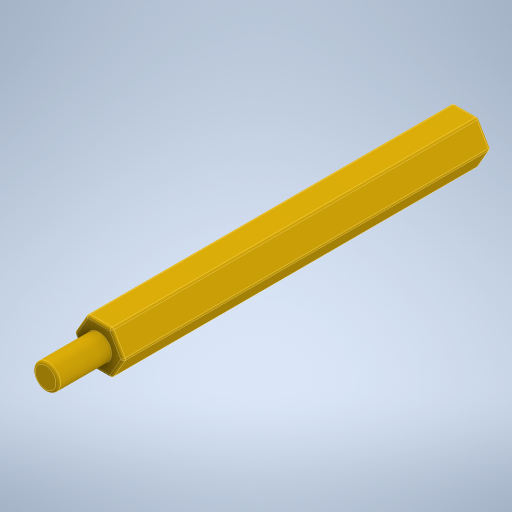
# Autodesk Inventor part: Espaciador_40mm
Saved by Autodesk Inventor 2023 (Build 270158030, 158C)
## iProperties
Created: 2022-07-21
Part Number: Espaciador_40mm
Material: Genérico
Document SubType Name: Modeling
Designer: luisn
Density: 1 g/cm^3
Appearance: Valor por defecto
Author: luisn
Autodesk Inventor part; units mm, degrees
ref_plane "YZ Plane" through (0, 0, 0) normal (1, 0, 0) x (0, 1, 0)
ref_plane "XZ Plane" through (0, 0, 0) normal (0, 1, 0) x (-1, 0, 0)
ref_plane "XY Plane" through (0, 0, 0) normal (0, 0, 1) x (1, 0, 0)
sketch "Boceto1" plane through (0, 0, 0) normal (0, 0, 1) x (1, 0, 0)
  line L0 (1.3423, 2.325) -> (2.6847, 0)
  line L1 (2.6847, 0) -> (1.3423, -2.325)
  line L2 (1.3423, -2.325) -> (-1.3423, -2.325)
  line L3 (-1.3423, -2.325) -> (-2.6847, 0)
  line L4 (-2.6847, 0) -> (-1.3423, 2.325)
  line L5 (-1.3423, 2.325) -> (1.3423, 2.325)
  point P0 (0, 0)
  point P1 (0, 0)
  point P2 (0, 0)
  dimension "d0" = 4.65
  constraints: 12 end point, 2 coincident, 1 horizontal, 13 other
  measures "d0" distance between parallel lines of L2 L5
extrude "Extrusión1" add sketch "Boceto1" along normal blind 40
sketch "Boceto2" plane through (0, 0, 40) normal (0, 0, 1) x (1, 0, 0)
  circle A0 centre (0, 0) radius 1.375
  dimension "d3" = 2.75
  constraints: 1 centre point, 1 coincident
  measures "d3" diameter of A0
extrude "Extrusión2" add sketch "Boceto2" along normal blind 5.8
fillet "Empalme1" radius 0.25 1 edges at (-1.375, 0, 45.8)
fillet "Empalme2" radius 0.25 18 edges at (-1.3423, 2.325, 20) (-2.6847, 0, 20) (1.3423, 2.325, 20) (2.6847, 0, 20) (1.3423, -2.325, 20) (-1.3423, -2.325, 20) (0, -2.325, 0) (-2.0135, -1.1625, 0) (-2.0135, 1.1625, 0) (2.0135, 1.1625, 0) (2.0135, -1.1625, 0) (0, 2.325, 0) (2.0135, -1.1625, 40) (0, -2.325, 40) (-2.0135, -1.1625, 40) (-2.0135, 1.1625, 40) (0, 2.325, 40) (2.0135, 1.1625, 40)
sketch "Boceto3" plane through (0, 0, 0) normal (0, 0, -1) x (-1, 0, 0)
  circle A0 centre (0, 0) radius 1.2
  dimension "d8" = 2.4
  constraints: 1 centre point, 1 coincident
  measures "d8" diameter of A0
extrude "Extrusión3" cut sketch "Boceto3" against normal blind 4
fillet "Empalme3" radius 0.25 1 edges at (1.2, 0, 0)
